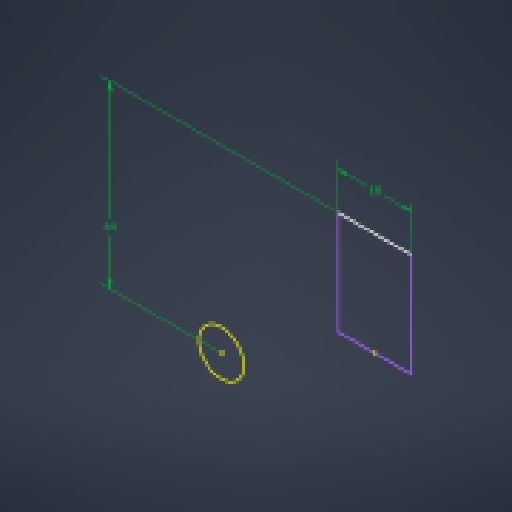
# Autodesk Inventor part: BandeV2Joint2
Saved by Autodesk Inventor 2026.3 (Build 303398000, 398)
## iProperties
Created: 2026-06-25
Part Number: BandeV2Joint2
Material: PET Plastic
Document SubType Name: Modeling
Designer: frede
Density: 1.541 g/cm^3
Appearance: White
Author: frede
Autodesk Inventor part; units mm, degrees
ref_plane "YZ Plane" through (0, 0, 0) normal (1, 0, 0) x (0, 1, 0)
ref_plane "XZ Plane" through (0, 0, 0) normal (0, 1, 0) x (-1, 0, 0)
ref_plane "XY Plane" through (0, 0, 0) normal (0, 0, 1) x (1, 0, 0)
sketch "Sketch1" plane through (0, 0, 0) normal (0, 0, 1) x (1, 0, 0)
  line L0 (-9, 0) -> (9, 0)
  line L1 (9, 0) -> (9, 50)
  line L2 (9, 50) -> (-9, 50)
  line L3 (-9, 50) -> (-9, 0)
  arc A0 (-2.25, 9) -> (2.25, 9) centre (0, 9) ccw
  arc A1 (2.25, 32) -> (-2.25, 32) centre (0, 32) ccw
  line L4 (-2.25, 32) -> (-2.25, 9)
  line L5 (2.25, 9) -> (2.25, 32)
  point P0 (0, 0)
  point P1 (0, 0)
  dimension "d0" = 18
  dimension "d2" = 4.5
  dimension "d3" = 50
  dimension "d4" = 4.5
  dimension "d7" = 18
  dimension "d8" = 9
  constraints: 12 end point, 4 point on circle, 3 tangent, 2 centre point, 2 horizontal, 2 parallel, 1 midpoint, 1 perpendicular
  measures "d0" distance of L2.end L1.end
  measures "d2" diameter of A0
  measures "d3" distance from line of point (0, 0) L2
  measures "d4" diameter of A1
  measures "d7" distance from line of L2 A1.centre
  measures "d8" distance from line of L0 A0.centre
extrude "Extrusion1" add sketch "Sketch1" along normal blind 5
sketch "Sketch2" plane through (0, 0, 0) normal (0, 0, -1) x (-1, 0, 0)
  line L0 (-9, 50) -> (9, 50) projected
  line L1 (9, 50) -> (9, 0) projected
  line L2 (-9, 50) -> (9, 50)
  line L3 (9, 50) -> (9, 45)
  line L4 (9, 45) -> (-9, 45)
  line L5 (-9, 45) -> (-9, 50)
  point P0 (0, 0)
  dimension "d9" = 5
  constraints: 8 end point, 2 parallel, 1 horizontal, 1 perpendicular, 1 point on line
  measures "d9" distance of L2.end L3.end
extrude "Extrusion2" add sketch "Sketch2" along normal blind 15
fillet "Fillet1" radius 2 1 edges at (0, 45, 0)
fillet "Fillet2" radius 7 1 edges at (0, 50, 5)
sketch "Sketch3" plane through (-9, 45, -15) normal (0, -1, 0) x (1, 0, 0)
  line L0 (0, 0) -> (18, 0) projected
  line L1 (0, 15) -> (18, 15) projected
  line L2 (0, 0) -> (18, 0)
  line L3 (18, 0) -> (18, 15)
  line L4 (18, 15) -> (0, 15)
  line L5 (0, 15) -> (0, 0)
  line L6 (18, 15) -> (0, 0)
  line L7 (6.9793, 4) -> (4.9585, 7.5)
  line L8 (4.9585, 7.5) -> (6.9793, 11)
  line L9 (6.9793, 11) -> (11.0207, 11)
  line L10 (11.0207, 11) -> (13.0415, 7.5)
  line L11 (13.0415, 7.5) -> (11.0207, 4)
  line L12 (11.0207, 4) -> (6.9793, 4)
  point P0 (9, 15)
  point P1 (9, 7.5)
  point P2 (9, 4)
  point P3 (11.7286, 9.7739)
  point P4 (6.2714, 5.2261)
  dimension "d14" = 7
  constraints: 22 end point, 2 midpoint, 2 parallel, 1 horizontal, 1 perpendicular, 13 other
  measures "d14" distance from line of point (9, 4) L9
extrude "Extrusion3" cut sketch "Sketch3" against normal blind 3.5 contours L7 L8 L9 L10 L6 | L6 L10 L11 L12 L7
sketch "Sketch4" plane through (-9, 48.5, -15) normal (0, -1, 0) x (1, 0, 0)
  line L0 (13.0415, 7.5) -> (11.0207, 4) projected
  line L1 (13.0415, 7.5) -> (4.9585, 7.5)
  circle A0 centre (9, 7.5) radius 2.2
  point P0 (9, 15)
  dimension "d17" = 4.4
  constraints: 2 end point, 1 centre point, 1 midpoint
  measures "d17" diameter of A0
extrude "Extrusion4" cut sketch "Sketch4" against normal up to surface (1.5 mm away)
sketch "Sketch6" plane through (-9, 50, -15) normal (0, 1, 0) x (1, 0, 0)
  line L0 (0, 0) -> (0, -13) projected
  line L1 (0, 0) -> (1.9, 0)
  line L2 (1.9, 0) -> (1.9, -18)
  line L3 (1.9, -18) -> (0, -18)
  line L4 (0, -18) -> (0, 0)
  line L5 (18, 0) -> (18, -13) projected
  line L6 (18, 0) -> (16.1, 0)
  line L7 (16.1, 0) -> (16.1, -18)
  line L8 (16.1, -18) -> (18, -18)
  line L9 (18, -18) -> (18, 0)
  point P0 (9, -15)
  dimension "d23" = 1.9
  dimension "d24" = 18
  dimension "d25" = 14.2
  dimension "d26" = 18
  constraints: 16 end point, 4 horizontal, 4 parallel, 2 perpendicular, 1 point on line
  measures "d23" distance between parallel lines of L2 L0
  measures "d24" distance between parallel lines of L5 L0
  measures "d25" distance between parallel lines of L7 L2
  measures "d26" distance between parallel lines of L1 L3
extrude "Extrusion5" add sketch "Sketch6" along normal blind 2 and the other way blind 5
fillet "Fillet4" radius 0.5 42 edges at (-2.2, 50, -7.5) (-2.2, 48.5, -7.5) (-3.0311, 45, -9.25) (0, 50, -15) (-7.1, 51, -15) (-8.05, 52, -15) (8.05, 52, -15) (7.1, 51, -15) (9, 48.5, -15) (0, 45, -15) (-9, 48.5, -15) (-7.1, 52, -6) (-9, 52, -6) (-8.05, 52, 3) (8.05, 52, 3) (7.1, 52, -6) (9, 52, -6) (9, 49.9495, 3) (7.1, 49.9495, 3) (-7.1, 49.9495, 3) (-9, 49.9495, 3) (9, 21.5, 5) (9, 45.6458, 4.4807) (-9, 21.5, 5) (-9, 45.6458, 4.4807) (0, 34.25, 5) (2.25, 20.5, 5) (0, 6.75, 5) (-2.25, 20.5, 5) (0, 34.25, 0) (2.25, 20.5, 0) (0, 6.75, 0) (-2.25, 20.5, 0) (9, 44.4142, -0.5858) (9, 45, -8.5) (9, 21.5, 0) (-9, 44.4142, -0.5858) (-9, 45, -8.5) (-9, 21.5, 0) (0, 0, 0) (-9, 0, 2.5) (9, 0, 2.5)
equation "\"d23\" = -0.5 * d25 + 0.5 * d24"
body "Solid1"
